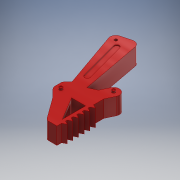
# Autodesk Inventor part: Part8
Saved by Autodesk Inventor 2022 (Build 260153000, 153)
## iProperties
Created: 2023-12-01
Part Number: Part8
Material: Generic
Document SubType Name: Modeling
Designer: harshidd
Density: 1 g/cm^3
Appearance: Red
Author: harshidd
Autodesk Inventor part; units mm, degrees
ref_plane "YZ Plane" through (0, 0, 0) normal (1, 0, 0) x (0, 1, 0)
ref_plane "XZ Plane" through (0, 0, 0) normal (0, 1, 0) x (-1, 0, 0)
sketch "Sketch1" plane through (0, 0, 0) normal (0, 0, 1) x (1, 0, 0)
  line L0 (0, 0) -> (-13.1942, 69.7633)
  line L1 (-13.1942, 69.7633) -> (-36.3853, 63.5848)
  line L2 (-36.3853, 63.5848) -> (-13.3296, -2.5093)
  line L3 (-13.3296, -2.5093) -> (-18.3981, -7.8428)
  line L4 (-18.3981, -7.8428) -> (-18.3981, -17.8428)
  line L5 (-18.3981, -17.8428) -> (-9.2098, -27.0392)
  line L6 (-9.2098, -27.0392) -> (8.4067, -51.3221)
  line L7 (8.4067, -51.3221) -> (19.4067, -51.3221)
  line L8 (19.4067, -51.3221) -> (19.4067, -1.3221)
  line L9 (19.4067, -1.3221) -> (23.6767, 7.7205)
  arc A0 (23.6767, 7.7205) -> (12.8256, 12.8444) centre (18.2512, 10.2824) ccw
  line L10 (8.5557, 3.8018) -> (12.8256, 12.8444)
  line L11 (0, 0) -> (8.5557, 3.8018)
  dimension "d0" = 71
  dimension "d1" = 24
  dimension "d2" = 70
  dimension "d3" = 20
  dimension "d4" = 10
  dimension "d5" = 13
  dimension "d6" = 30
  dimension "d8" = 11
  dimension "d9" = 50
  dimension "d10" = 10
  dimension "d11" = 12
  dimension "d12" = 10
  constraints: 24 end point, 2 point on circle, 2 tangent, 1 centre point, 1 horizontal, 1 parallel, 1 perpendicular, 1 vertical
  measures "d0" distance of L0.start L0.end
  measures "d1" distance of L0.end L1.end
  measures "d2" distance of L2.end L1.end
  measures "d3" distance of L0.start L3.end
  measures "d4" distance of L3.end L4.end
  measures "d5" distance of L4.end L5.end
  measures "d6" distance of L5.end L6.end
  measures "d8" distance of L6.end L7.end
  measures "d9" distance of L7.end L8.end
  measures "d10" distance of L8.end L9.end
  measures "d11" distance of L9.end L10.end
  measures "d12" distance of L10.end L10.start
extrude "Extrusion1" add sketch "Sketch1" along normal blind 18
sketch "Sketch2" plane through (0, 0, 18) normal (0, 0, 1) x (1, 0, 0)
  line L0 (16.2045, -42.4982) -> (16.2045, -17.4982)
  line L1 (16.2045, -17.4982) -> (1.2045, -17.4982)
  line L2 (1.2045, -17.4982) -> (16.2045, -42.4982)
  point P0 (0, 0)
  dimension "d15" = 25
  dimension "d16" = 15
  constraints: 6 end point, 1 perpendicular, 1 vertical
  measures "d15" distance of L0.start L0.end
  measures "d16" distance of L0.end L1.end
extrude "Extrusion2" cut sketch "Sketch2" against normal blind 18
sketch "Sketch3" plane through (0, 0, 18) normal (0, 0, 1) x (1, 0, 0)
  line L0 (19.4067, -51.3221) -> (19.4067, -1.3221) construction
  line L1 (19.4067, -51.3221) -> (19.4067, -46.3221) construction
  line L2 (19.4067, -46.3221) -> (19.4067, -42.3221)
  line L3 (19.4067, -44.3221) -> (23.4067, -44.3221) construction
  line L4 (19.4067, -42.3221) -> (23.4067, -44.3221)
  line L5 (19.4067, -46.3221) -> (23.4067, -44.3221)
  point P0 (0, 0)
  dimension "d19" = 5
  dimension "d20" = 4
  dimension "d21" = 4
  constraints: 10 end point, 2 point on line, 1 horizontal, 1 midpoint
  measures "d19" distance of L0.start L1.end
  measures "d20" distance of L1.end L2.end
  measures "d21" distance of L3.start L3.end
extrude "Extrusion3" add sketch "Sketch3" against normal blind 18
pattern_linear "Rectangular Pattern1" count 6 spacing 6 along (0, 1, 0) of "Extrusion3"
fillet "Fillet1" radius 6 3 edges at (-18.3981, -17.8428, 9) (-36.3853, 63.5848, 9) (-13.1942, 69.7633, 9)
fillet "Fillet2" radius 4 2 edges at (-18.3981, -7.8428, 9) (8.4067, -51.3221, 9)
sketch "Sketch5" plane through (0, 0, 18) normal (0, 0, 1) x (1, 0, 0)
  arc A0 (-30.1339, 65.2503) -> (-34.2545, 57.4763) centre (-28.5892, 59.4525) ccw projected
  circle A1 centre (-28.5892, 59.4525) radius 1.5
  point P0 (0, 0)
  dimension "d32" = 3
  constraints: 1 centre point, 1 coincident
  measures "d32" diameter of A1
extrude "Extrusion5" cut sketch "Sketch5" against normal blind 18
sketch "Sketch6" plane through (-9.2098, -27.0392, 0) normal (-0.8094, -0.5872, 0) x (0, 0, 1)
  line L0 (3, -3) -> (15, -3)
  line L1 (0, 0) -> (0, -27.9601) projected
  line L2 (18, 0) -> (18, -27.9601) projected
  line L3 (0, 0) -> (18, 0) projected
  line L4 (3, -3) -> (4.5418, -23.4291)
  line L5 (18, -23.4291) -> (0, -23.4291) projected
  line L6 (15, -3) -> (13.4582, -23.4291)
  point P0 (0, 16.4781)
  dimension "d35" = 3
  dimension "d36" = 3
  dimension "d37" = 3
  constraints: 6 end point, 2 point on line, 1 equal length
  measures "d35" distance from line of L1 L0.start
  measures "d36" distance from line of L2 L0.end
  measures "d37" distance between parallel lines of L3 L0
extrude "Extrusion6" cut sketch "Sketch6" against normal blind 14 contours L0 L6 L5 L4
sketch "Sketch7" plane through (0, 0, 18) normal (0, 0, 1) x (1, 0, 0)
  arc A0 (-18.3981, -15.359) -> (-16.6426, -19.5998) centre (-12.3981, -15.359) ccw projected
  circle A1 centre (-12.3981, -15.359) radius 1.75
  arc A2 (23.6767, 7.7205) -> (12.8256, 12.8444) centre (18.2512, 10.2824) ccw projected
  circle A3 centre (18.2512, 10.2824) radius 1.75
  point P0 (0, 0)
  dimension "d40" = 3.5
  dimension "d41" = 3.5
  constraints: 2 centre point, 2 coincident
  measures "d40" diameter of A1
  measures "d41" diameter of A3
extrude "Extrusion7" add sketch "Sketch7" along normal blind 2
sketch "Sketch9" plane through (18.2512, 10.2824, 20) normal (0, 0, 1) x (1, 0, 0)
  circle A0 centre (0, 0) radius 1.75 projected
  circle A1 centre (-30.6493, -25.6415) radius 1.75 projected
  circle A2 centre (0, 0) radius 1.25
  circle A3 centre (-30.6493, -25.6415) radius 1.25
  point P0 (-18.2512, -10.2824)
  dimension "d44" = 0.5
  dimension "d45" = 0.5
  constraints: 2 centre point
  measures "d44" radial gap between concentric circles of A0 A2
  measures "d45" radial gap between concentric circles of A1 A3
extrude "Extrusion8" cut sketch "Sketch9" against normal blind 0.5 contours A2 | A3
sketch "Sketch10" plane through (0, 0, 18) normal (0, 0, 1) x (1, 0, 0)
  line L0 (-21.8945, 53.635) -> (-10.3211, 10.7097) construction
  line L1 (-24.5497, 52.9192) -> (-12.9763, 9.9938)
  line L2 (-7.6659, 11.4256) -> (-19.2393, 54.3509)
  arc A0 (-19.2393, 54.3509) -> (-24.5497, 52.9192) centre (-21.8945, 53.635) ccw
  arc A1 (-12.9763, 9.9938) -> (-7.6659, 11.4256) centre (-10.3211, 10.7097) ccw
  point P0 (0, 0)
  point P1 (-16.1078, 32.1724)
  dimension "d48" = 5.5
  constraints: 8 end point, 4 point on circle, 4 tangent, 2 centre point, 1 midpoint, 1 parallel
  measures "d48" diameter of A1
extrude "Extrusion9" cut sketch "Sketch10" against normal blind 1
ref_plane "Work Plane1" through (0, 0, 9) normal (0, 0, 1) x (1, 0, 0)
mirror "Mirror1" about plane through (0, 0, 9) normal (0, 0, 1) of "Extrusion9", "Extrusion7", "Extrusion8"
body "Solid1"
